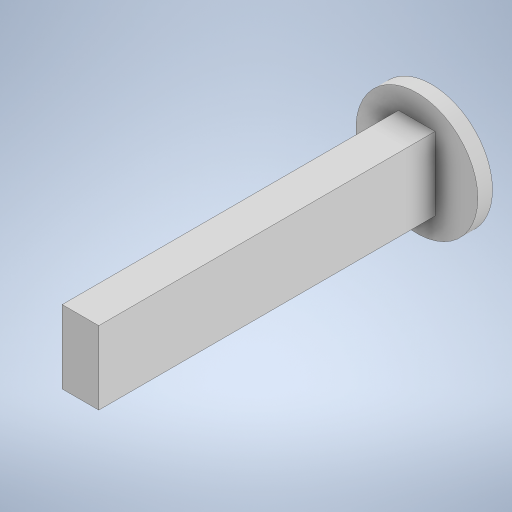
# Autodesk Inventor part: NHK_t0_5
Saved by Autodesk Inventor 2023 (Build 270158000, 158)
## iProperties
Created: 2022-04-19
Part Number: NHK_t0_5
Material: 一般
Document SubType Name: Modeling
Designer: yuta
Density: 1 g/cm^3
Appearance: 既定
Author: yuta
Autodesk Inventor part; units mm, degrees
ref_plane "YZ Plane" through (0, 0, 0) normal (1, 0, 0) x (0, 1, 0)
ref_plane "XZ Plane" through (0, 0, 0) normal (0, 1, 0) x (-1, 0, 0)
ref_plane "XY Plane" through (0, 0, 0) normal (0, 0, 1) x (1, 0, 0)
sketch "スケッチ1" plane through (0, 0, 0) normal (0, 0, 1) x (1, 0, 0)
  circle A0 centre (0, 0) radius 25
  dimension "d0" = 50
  constraints: 1 centre point, 1 coincident
  measures "d0" diameter of A0
extrude "押し出し1" add sketch "スケッチ1" along normal blind 6
sketch "スケッチ2" plane through (0, 0, 6) normal (0, 0, 1) x (1, 0, 0)
  line L0 (-7.5, 15) -> (7.5, 15)
  line L1 (7.5, 15) -> (7.5, -15)
  line L2 (7.5, -15) -> (-7.5, -15)
  line L3 (-7.5, -15) -> (-7.5, 15)
  circle A0 centre (0, 0) radius 25 projected
  dimension "d3" = 15
  dimension "d4" = 30
  dimension "d5" = 7.5
  dimension "d6" = 15
  constraints: 8 end point, 2 parallel, 1 horizontal, 1 perpendicular
  measures "d3" distance of L1.end L2.end
  measures "d4" distance of L0.end L1.end
  measures "d5" distance from line of L3 A0.centre
  measures "d6" distance from line of point (0, 0) L2
extrude "押し出し2" add sketch "スケッチ2" along normal blind 100 contours L0 L1 L2 L3
sketch "スケッチ3" plane through (0, 0, 106) normal (0, 0, 1) x (1, 0, 0)
  circle A0 centre (0, 0) radius 25
  dimension "d9" = 50
  constraints: 1 centre point, 1 coincident
  measures "d9" diameter of A0
extrude "押し出し3" cut sketch "スケッチ3" against normal blind 6
sketch "スケッチ4" plane through (0, 0, 100) normal (0, 0, 1) x (1, 0, 0)
  circle A0 centre (0, 0) radius 25
  dimension "d12" = 50
  constraints: 1 centre point, 1 coincident
  measures "d12" diameter of A0
extrude "押し出し4" add sketch "スケッチ4" along normal blind 6
sketch "スケッチ5" plane through (0, 0, 106) normal (0, 0, 1) x (1, 0, 0)
  circle A0 centre (0, 0) radius 25
  dimension "d15" = 50
  constraints: 1 centre point, 1 coincident
  measures "d15" diameter of A0
extrude "押し出し5" cut sketch "スケッチ5" against normal blind 6
sketch "スケッチ6" plane through (0, 0, 100) normal (0, 0, 1) x (1, 0, 0)
  line L0 (-7.5, -15) -> (-7.5, 15) projected
  line L1 (-7.5, 15) -> (7.5, 15) projected
  line L2 (-7.5, -15) -> (7.5, -15)
  line L3 (7.5, -15) -> (7.5, 15)
  line L4 (7.5, 15) -> (-7.5, 15)
  line L5 (-7.5, 15) -> (-7.5, -15)
  point P0 (0, 0)
  constraints: 8 end point, 2 parallel, 1 horizontal, 1 perpendicular
extrude "押し出し6" add sketch "スケッチ6" along normal blind 44
sketch "スケッチ7" plane through (0, 0, 144) normal (0, 0, 1) x (1, 0, 0)
  circle A0 centre (0, 0) radius 25
  dimension "d20" = 50
  constraints: 1 centre point, 1 coincident
  measures "d20" diameter of A0
extrude "押し出し7" add sketch "スケッチ7" along normal blind 6
sketch "スケッチ8" plane through (0, 0, 150) normal (0, 0, 1) x (1, 0, 0)
  circle A0 centre (0, 0) radius 25
  dimension "d23" = 50
  constraints: 1 centre point, 1 coincident
  measures "d23" diameter of A0
extrude "押し出し8" cut sketch "スケッチ8" against normal blind 6
